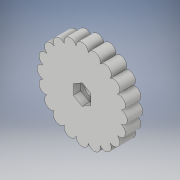
# Autodesk Inventor part: 00_gear
Saved by Autodesk Inventor 2019 (Build 230136000, 136)
## iProperties
Created: 2020-06-16
Part Number: 00_gear
Material: Generic
Document SubType Name: Modeling
Designer: UC2
Density: 1 g/cm^3
Appearance: Default
Author: UC2
Autodesk Inventor part; units mm, degrees
ref_plane "YZ Plane" through (0, 0, 0) normal (1, 0, 0) x (0, 1, 0)
ref_plane "XZ Plane" through (0, 0, 0) normal (0, 1, 0) x (-1, 0, 0)
ref_plane "XY Plane" through (0, 0, 0) normal (0, 0, 1) x (1, 0, 0)
sketch "Skizze1" plane through (0, 0, 0) normal (0, 0, 1) x (1, 0, 0)
  line L0 (-20.3, 0) -> (20.3, 0) construction
  line L1 (0, -20.3) -> (0, 20.3) construction
  circle A0 centre (0, 0) radius 12.5
  circle A1 centre (0, 0) radius 1.6
  arc A2 (1.9936, 12.34) -> (-1.9936, 12.34) centre (0, 12.5) ccw
  circle A3 centre (0, 0) radius 14.5 construction
  dimension "d1" = 3.2
  dimension "d2" = 2
  dimension "d3" = 29
  constraints: 5 point on circle, 4 centre point, 3 coincident, 1 point on line, 1 tangent
  measures "d1" diameter of A1
  measures "d2" radius of A2
  measures "d3" diameter of A3
extrude "Extrusion1" add sketch "Skizze1" along normal blind 5
pattern_circular "Runde Anordnung1" count 20 over 360 about axis through (0, 0, -10) along (0, 0, 1) of "Extrusion1"
sketch "Skizze2" plane through (0, 0, 5) normal (0, 0, 1) x (1, 0, 0)
  circle A0 centre (0, 0) radius 1.6 construction
  arc A1 (-1.997, 12.6088) -> (-5.7956, 11.3746) centre (-3.8627, 11.8882) ccw construction
  arc A2 (-5.7956, 11.3746) -> (-9.0269, 9.0269) centre (-7.3473, 10.1127) ccw construction
  arc A3 (-9.0269, 9.0269) -> (-11.3746, 5.7956) centre (-10.1127, 7.3473) ccw construction
  arc A4 (-11.3746, 5.7956) -> (-12.6088, 1.997) centre (-11.8882, 3.8627) ccw construction
  arc A5 (-12.6088, 1.997) -> (-12.6088, -1.997) centre (-12.5, 0) ccw construction
  arc A6 (-12.6088, -1.997) -> (-11.3746, -5.7956) centre (-11.8882, -3.8627) ccw construction
  arc A7 (-11.3746, -5.7956) -> (-9.0269, -9.0269) centre (-10.1127, -7.3473) ccw construction
  arc A8 (-9.0269, -9.0269) -> (-5.7956, -11.3746) centre (-7.3473, -10.1127) ccw construction
  arc A9 (-5.7956, -11.3746) -> (-1.997, -12.6088) centre (-3.8627, -11.8882) ccw construction
  arc A10 (-1.997, -12.6088) -> (1.997, -12.6088) centre (0, -12.5) ccw construction
  arc A11 (1.997, -12.6088) -> (5.7956, -11.3746) centre (3.8627, -11.8882) ccw construction
  arc A12 (5.7956, -11.3746) -> (9.0269, -9.0269) centre (7.3473, -10.1127) ccw construction
  arc A13 (9.0269, -9.0269) -> (11.3746, -5.7956) centre (10.1127, -7.3473) ccw construction
  arc A14 (11.3746, -5.7956) -> (12.6088, -1.997) centre (11.8882, -3.8627) ccw construction
  arc A15 (12.6088, -1.997) -> (12.6088, 1.997) centre (12.5, 0) ccw construction
  arc A16 (12.6088, 1.997) -> (11.3746, 5.7956) centre (11.8882, 3.8627) ccw construction
  arc A17 (11.3746, 5.7956) -> (9.0269, 9.0269) centre (10.1127, 7.3473) ccw construction
  arc A18 (9.0269, 9.0269) -> (5.7956, 11.3746) centre (7.3473, 10.1127) ccw construction
  arc A19 (5.7956, 11.3746) -> (1.997, 12.6088) centre (3.8627, 11.8882) ccw construction
  arc A20 (1.997, 12.6088) -> (-1.997, 12.6088) centre (0, 12.5) ccw construction
  line L0 (-20.3, 0) -> (20.3, 0) construction
  line L1 (0, -20.3) -> (0, 20.3) construction
  line L2 (0, 3.25) -> (2.8146, 1.625)
  line L3 (2.8146, 1.625) -> (2.8146, -1.625)
  line L4 (2.8146, -1.625) -> (0, -3.25)
  line L5 (0, -3.25) -> (-2.8146, -1.625)
  line L6 (-2.8146, -1.625) -> (-2.8146, 1.625)
  line L7 (-2.8146, 1.625) -> (0, 3.25)
  dimension "d9" = 6.5
  constraints: 12 end point, 1 coincident, 1 point on line, 13 other
  measures "d9" distance of L4.end L2.start
extrude "Extrusion2" cut sketch "Skizze2" against normal blind 2.4
